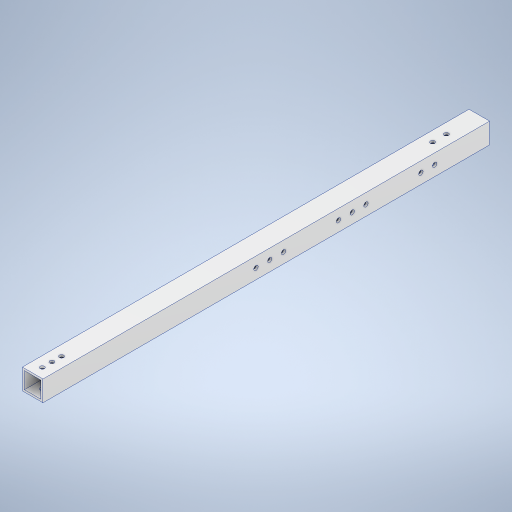
# Autodesk Inventor part: 射出_角柱4
Saved by Autodesk Inventor 2023 (Build 270158000, 158)
## iProperties
Created: 2022-04-20
Part Number: 射出_角柱4
Material: アルミニウム 6061
Document SubType Name: Modeling
Designer: yuta
Density: 2.7 g/cm^3
Appearance: アルミニウム - フラット
Author: yuta
Autodesk Inventor part; units mm, degrees
ref_plane "YZ Plane" through (0, 0, 0) normal (1, 0, 0) x (0, 1, 0)
ref_plane "XZ Plane" through (0, 0, 0) normal (0, 1, 0) x (-1, 0, 0)
ref_plane "XY Plane" through (0, 0, 0) normal (0, 0, 1) x (1, 0, 0)
sketch "スケッチ1" plane through (0, 0, 0) normal (0, 0, 1) x (1, 0, 0)
  line L0 (0, 0) -> (15, 0)
  line L1 (15, 0) -> (15, 15)
  line L2 (15, 15) -> (0, 15)
  line L3 (0, 15) -> (0, 0)
  dimension "d0" = 15
  dimension "d1" = 15
  constraints: 8 end point, 2 parallel, 1 horizontal, 1 perpendicular
  measures "d0" distance of L2.end L1.end
  measures "d1" distance of L1.end L0.end
extrude "押し出し1" add sketch "スケッチ1" along normal blind 140
sketch "スケッチ3" plane through (0, 0, 0) normal (0, 0, -1) x (-1, 0, 0)
  line L0 (0, 0) -> (-15, 0)
  line L1 (-15, 0) -> (-15, 15)
  line L2 (-15, 15) -> (0, 15)
  line L3 (0, 15) -> (0, 0)
  dimension "d18" = 15
  dimension "d19" = 15
  constraints: 8 end point, 2 parallel, 1 horizontal, 1 perpendicular
  measures "d18" distance of L1.end L2.end
  measures "d19" distance of L0.end L1.end
extrude "押し出し2" add sketch "スケッチ3" along normal blind 200
sketch "スケッチ4" plane through (0, 0, -200) normal (0, 0, -1) x (-1, 0, 0)
  point P0 (0, 0)
sketch "スケッチ6" plane through (0, 0, 140) normal (0, 0, 1) x (1, 0, 0)
  line L0 (0, 0) -> (0, 15) projected
  line L1 (15, 15) -> (15, 0) projected
  line L2 (0, 0) -> (15, 0)
  line L3 (15, 0) -> (15, 15)
  line L4 (15, 15) -> (0, 15)
  line L5 (0, 15) -> (0, 0)
  constraints: 8 end point, 2 parallel, 1 horizontal, 1 perpendicular
extrude "押し出し3" cut sketch "スケッチ6" against normal blind 15
sketch "スケッチ8" plane through (0, 15, -200) normal (0, 1, 0) x (1, 0, 0)
  line L0 (0, 0) -> (15, 0) projected
  line L1 (15, 0) -> (15, -325) projected
  point P0 (0, -200)
  point P1 (7.5, -24)
  dimension "d36" = 24
  dimension "d37" = 7.5
  measures "d36" distance from line of L0 point (7.5, -24)
  measures "d37" distance from line of L1 point (7.5, -24)
hole "穴3" at (7.5, 15, -176) direction (0, -1, 0) diameter 3.2 end through all
sketch "スケッチ9" plane through (15, 0, -200) normal (1, 0, 0) x (0, 0, -1)
  line L0 (0, 15) -> (0, 0) projected
  line L1 (0, 15) -> (-325, 15) projected
  line L2 (-325, 0) -> (0, 0) projected
  point P0 (-200, 0)
  point P1 (-90, 7.5)
  point P2 (-100, 7.5)
  point P3 (-110, 7.5)
  point P4 (-150, 7.5)
  point P5 (-160, 7.5)
  point P6 (-170, 7.5)
  dimension "d45" = 90
  dimension "d46" = 7.5
  dimension "d47" = 10
  dimension "d48" = 10
  dimension "d49" = 7.5
  dimension "d50" = 7.5
  dimension "d51" = 40
  dimension "d52" = 7.5
  dimension "d53" = 10
  dimension "d54" = 7.5
  dimension "d55" = 10
  dimension "d56" = 7.5
  measures "d45" distance from line of L0 point (-90, 7.5)
  measures "d46" distance from line of L1 point (-90, 7.5)
  measures "d47" distance of point (-90, 7.5) point (-100, 7.5)
  measures "d48" distance of point (-110, 7.5) point (-100, 7.5)
  measures "d49" distance from line of L2 point (-100, 7.5)
  measures "d50" distance from line of L2 point (-110, 7.5)
  measures "d51" distance of point (-110, 7.5) point (-150, 7.5)
  measures "d52" distance from line of L2 point (-150, 7.5)
  measures "d53" distance of point (-150, 7.5) point (-160, 7.5)
  measures "d54" distance from line of L2 point (-160, 7.5)
  measures "d55" distance of point (-160, 7.5) point (-170, 7.5)
  measures "d56" distance from line of L2 point (-170, 7.5)
hole "穴4" at (15, 7.5, -30) at (15, 7.5, -40) at (15, 7.5, -50) at (15, 7.5, -90) at (15, 7.5, -100) at (15, 7.5, -110) direction (-1, 0, 0) diameter 3.2 end through all
sketch "スケッチ10" plane through (0, 15, -200) normal (0, 1, 0) x (1, 0, 0)
  circle A0 centre (7.5, -24) radius 1.6 projected
  line L0 (15, 0) -> (15, -325) projected
  point P0 (0, -200)
  point P1 (7.5, -34)
  dimension "d64" = 10
  dimension "d65" = 7.5
  measures "d64" distance of point (7.5, -34) A0.centre
  measures "d65" distance from line of L0 point (7.5, -34)
hole "穴5" at (7.5, 15, -166) direction (0, -1, 0) diameter 3.2 end through all
sketch "スケッチ11" plane through (0, 15, -200) normal (0, 1, 0) x (1, 0, 0)
  line L0 (0, -325) -> (15, -325) projected
  line L1 (15, 0) -> (15, -325) projected
  point P0 (0, -200)
  point P1 (7.5, -318)
  point P2 (7.5, -311)
  point P3 (7.5, -304)
  dimension "d73" = 7
  dimension "d74" = 7.5
  dimension "d75" = 7
  dimension "d76" = 7.5
  dimension "d77" = 7
  dimension "d78" = 7.5
  measures "d73" distance from line of L0 point (7.5, -318)
  measures "d74" distance from line of L1 point (7.5, -318)
  measures "d75" distance of point (7.5, -318) point (7.5, -311)
  measures "d76" distance from line of L1 point (7.5, -311)
  measures "d77" distance of point (7.5, -311) point (7.5, -304)
  measures "d78" distance from line of L1 point (7.5, -304)
hole "穴6" at (7.5, 15, 111) at (7.5, 15, 118) at (7.5, 15, 104) direction (0, -1, 0) diameter 3.2 end through all
sketch "スケッチ12" plane through (15, 0, -200) normal (1, 0, 0) x (0, 0, -1)
  line L0 (0, 15) -> (0, 0) projected
  line L1 (-325, 0) -> (0, 0) projected
  line L2 (0, 15) -> (-325, 15) projected
  point P0 (-200, 0)
  point P1 (-40, 7.5)
  point P2 (-50, 7.5)
  dimension "d86" = 40
  dimension "d87" = 7.5
  dimension "d88" = 7.5
  dimension "d89" = 10
  measures "d86" distance from line of L0 point (-40, 7.5)
  measures "d87" distance from line of L1 point (-40, 7.5)
  measures "d88" distance from line of L2 point (-50, 7.5)
  measures "d89" distance of point (-40, 7.5) point (-50, 7.5)
hole "穴7" at (15, 7.5, -150) at (15, 7.5, -160) direction (-1, 0, 0) diameter 3.2 end through all
sketch "スケッチ13" plane through (0, 0, 125) normal (0, 0, 1) x (1, 0, 0)
  line L0 (1.5, 13.5) -> (13.5, 13.5)
  line L1 (13.5, 13.5) -> (13.5, 1.5)
  line L2 (13.5, 1.5) -> (1.5, 1.5)
  line L3 (1.5, 1.5) -> (1.5, 13.5)
  line L4 (0, 15) -> (15, 15) projected
  line L5 (0, 0) -> (0, 15) projected
  dimension "d97" = 12
  dimension "d98" = 12
  dimension "d99" = 1.5
  dimension "d100" = 1.5
  constraints: 8 end point, 2 parallel, 1 horizontal, 1 perpendicular
  measures "d97" distance of L1.end L2.end
  measures "d98" distance of L0.end L1.end
  measures "d99" distance between parallel lines of L4 L0
  measures "d100" distance between parallel lines of L5 L3
extrude "押し出し4" cut sketch "スケッチ13" against normal blind 450
